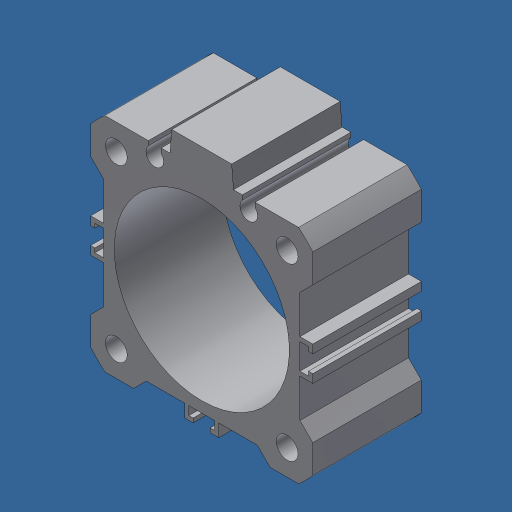
# Autodesk Inventor part: EXTRUSION, CYLINDER, ALUMINIUM, SMC, 40MM
Saved by Autodesk Inventor 2024.3 (Build 283343000, 343)
## iProperties
ILogicPurgeVersion: 2.2.20.20
Category: _
Manager: _
Shininess: 64.0
Angle Display Precision: 2
Document Length Units: 11272
Document Angle Units: 11279
Document Time Units: 11290
Document Mass Units: 11286
Document Length Units Precision: 3
Document Angle Units Precision: 2
Part Number: EXTRUSION, CYLINDER, ALUMINIUM, SMC, 40MM
Material: Extrusion, Aluminum, SMC, 40 MM
Document SubType Name: Modeling
Created: 2019-07-31
Designer: -
Manufacturer: Standard
Standards Organization: Custom
Density: 2.71 g/cm^3
Mass: 74.6962 g
Surface Area: 142.466 cm^2
Volume: 27.5632 cm^3
Checked By: 00
Engr Approved By: _
User Status: Work In Process
Description: EXTRUSION, CYLINDER, ALUMINIUM, SMC, 40MM
Mfg Approved By: -
Appearance: Aluminum - Flat
Density: 0.0
Volumn: 0.0
Area: 0.0
PropertySet Name: Model Information
Control State: 0
Master: False
Checked Out: False
CN_MASS: 0.07
CN_SERVICEABLE: _
CL_runCount: 0
FIRST_DESCRIPTION: _
SECOND_DESCRIPTION: _
THIRD_DESCRIPTION: _
ModelCat: Uncategorized
Author: -
Subject: _
Revision Number: A
Keywords: -
Autodesk Inventor part; units mm, degrees
ref_plane "YZ Plane" through (0, 0, 0) normal (1, 0, 0) x (0, 1, 0)
ref_plane "XZ Plane" through (0, 0, 0) normal (0, 1, 0) x (-1, 0, 0)
ref_plane "XY Plane" through (0, 0, 0) normal (0, 0, 1) x (1, 0, 0)
sketch "Sketch1" plane through (0, 0, 0) normal (0, 0, 1) x (1, 0, 0)
  line L0 (-7.4374, 26) -> (-7, 31)
  line L1 (0, 31) -> (0, 0) construction
  line L2 (-7, 31) -> (0, 31)
  line L3 (-9.5, 26) -> (-9.5, 24.9337)
  line L4 (-12.5, 26) -> (-12.5, 24.9337)
  line L5 (-7.4374, 26) -> (-9.5, 26)
  line L6 (-12.5, 26) -> (-22.6771, 26)
  arc A0 (-12.5, 24.9337) -> (-9.5, 24.9337) centre (-11, 23.5) ccw
  line L7 (-22.6771, -26) -> (-16, -26)
  line L8 (0, -23) -> (0, 0) construction
  arc A1 (-26, -22.6771) -> (-22.6771, -26) centre (0, 0) ccw
  arc A2 (-22.6771, 26) -> (-26, 22.6771) centre (0, 0) ccw
  line L9 (-26, 16) -> (-23, 13)
  line L10 (-23, -13) -> (-26, -16)
  line L11 (-26, 22.6771) -> (-26, 16)
  line L12 (-26, -16) -> (-26, -22.6771)
  line L13 (-16, -26) -> (-13, -23)
  line L14 (-23, 4) -> (-26, 4)
  line L15 (-26, 4) -> (-26, 2)
  line L16 (-26, 2) -> (-25, 2)
  line L17 (-25, 2) -> (-25, 3)
  line L18 (-25, 3) -> (-23, 3)
  line L19 (-23, -4) -> (-26, -4)
  line L20 (-26, -4) -> (-26, -2)
  line L21 (-26, -2) -> (-25, -2)
  line L22 (-25, -2) -> (-25, -3)
  line L23 (-25, -3) -> (-23, -3)
  line L24 (-4, -23) -> (-4, -26)
  line L25 (-4, -26) -> (-2, -26)
  line L26 (-2, -26) -> (-2, -25)
  line L27 (-2, -25) -> (-3, -25)
  line L28 (-3, -25) -> (-3, -23)
  line L29 (-23, 13) -> (-23, 4)
  line L30 (-23, 3) -> (-23, -3)
  line L31 (-23, -4) -> (-23, -13)
  line L32 (-13, -23) -> (-4, -23)
  line L33 (-3, -23) -> (0, -23)
  arc A3 (0, 20.5) -> (0, -20.5) centre (0, 0) ccw
  line L34 (0, 36.125) -> (0, -43.6282) construction
  line L35 (7.4374, 26) -> (7, 31)
  line L36 (7, 31) -> (0, 31)
  line L37 (9.5, 26) -> (9.5, 24.9337)
  line L38 (12.5, 26) -> (12.5, 24.9337)
  line L39 (7.4374, 26) -> (9.5, 26)
  line L40 (12.5, 26) -> (22.6771, 26)
  arc A4 (9.5, 24.9337) -> (12.5, 24.9337) centre (11, 23.5) ccw
  line L41 (22.6771, -26) -> (16, -26)
  arc A5 (22.6771, -26) -> (26, -22.6771) centre (0, 0) ccw
  arc A6 (26, 22.6771) -> (22.6771, 26) centre (0, 0) ccw
  line L42 (26, 16) -> (23, 13)
  line L43 (23, -13) -> (26, -16)
  line L44 (26, 22.6771) -> (26, 16)
  line L45 (26, -16) -> (26, -22.6771)
  line L46 (16, -26) -> (13, -23)
  line L47 (23, 4) -> (26, 4)
  line L48 (26, 4) -> (26, 2)
  line L49 (26, 2) -> (25, 2)
  line L50 (25, 2) -> (25, 3)
  line L51 (25, 3) -> (23, 3)
  line L52 (23, -4) -> (26, -4)
  line L53 (26, -4) -> (26, -2)
  line L54 (26, -2) -> (25, -2)
  line L55 (25, -2) -> (25, -3)
  line L56 (25, -3) -> (23, -3)
  line L57 (4, -23) -> (4, -26)
  line L58 (4, -26) -> (2, -26)
  line L59 (2, -26) -> (2, -25)
  line L60 (2, -25) -> (3, -25)
  line L61 (3, -25) -> (3, -23)
  line L62 (23, 13) -> (23, 4)
  line L63 (23, 3) -> (23, -3)
  line L64 (23, -4) -> (23, -13)
  line L65 (13, -23) -> (4, -23)
  line L66 (3, -23) -> (0, -23)
  arc A7 (0, -20.5) -> (0, 20.5) centre (0, 0) ccw
  point P0 (-20, 20)
  point P1 (-20, -20)
  point P2 (20, 20)
  point P3 (20, -20)
  dimension "d3" = 7.4374
  dimension "d4" = 7
  dimension "d6" = 31
  dimension "d7" = 5
  dimension "d8" = 3
  dimension "d9" = 2.075
  dimension "d10" = 2.5
  dimension "d11" = 11
  dimension "d15" = 34.5
  dimension "d16" = 34.5
  dimension "d19" = 26
  dimension "d20" = 13
  dimension "d21" = 26
  dimension "d22" = 26
  dimension "d23" = 6.6771
  dimension "d24" = 23
  dimension "d25" = 1
  dimension "d26" = 1
  dimension "d27" = 26
  dimension "d28" = 8
  dimension "d29" = 4
  dimension "d30" = 4
  dimension "d31" = 2
  dimension "d32" = 20.5
  dimension "d33" = 40
  dimension "d34" = 20
  dimension "d35" = 20
  constraints: 134 end point, 37 symmetric about line, 22 perpendicular, 19 parallel, 16 point on circle, 13 equal length, 8 centre point, 3 coincident, 3 vertical alignment, 2 horizontal, 2 horizontal alignment, 2 point on line, 36 other
  measures "d3" horizontal distance of L1.end L0.start
  measures "d4" distance of L0.end L1.start
  measures "d6" distance of L1.start L1.end
  measures "d7" distance between parallel lines of L5 L2
  measures "d8" distance between parallel lines of L3 L4
  measures "d9" radius of A0
  measures "d10" distance from line of L5 A0.centre
  measures "d11" distance from line of L1 A0.centre
  measures "d15" radius of A2
  measures "d16" radius of A1
  measures "d19" distance of L9.end L10.start
  measures "d20" vertical distance of L1.end L9.end
  measures "d21" distance between parallel lines of L1 L11
  measures "d22" distance from line of L7 L1.end
  measures "d23" distance of L7.start L7.end
  measures "d24" distance from line of L1.end L33
  measures "d25" distance of L15.end L16.end
  measures "d26" distance between parallel lines of L14 L18
  measures "d27" distance from line of L1.end L20
  measures "d28" distance between parallel lines of L19 L14
  measures "d29" distance between parallel lines of L8 L24
  measures "d30" distance from line of L1.end L19
  measures "d31" distance of L19.end L20.end
  measures "d32" radius of A3
  measures "d33" distance of point (-20, -20) point (-20, 20)
  measures "d34" horizontal distance of point (-20, -20) L1.end
  measures "d35" distance from line of L1 point (-20, 20)
extrude "SMC, 40MM" add sketch "Sketch1" along normal blind 25.4
hole "Hole1" at (-20, 20, 0) at (-20, -20, 0) at (20, 20, 0) at (20, -20, 0) direction (0, 0, 1) diameter 5.1054 end through all
equation "\"d20\" = 0.5 * d19"
equation "\"d26\" = d25"
equation "\"d30\" = 0.5 * d28"
equation "\"d34\" = 0.5 * d33"
equation "\"d35\" = d34"
